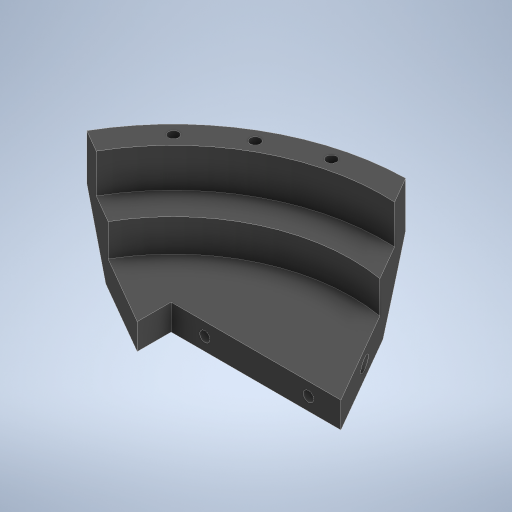
# Autodesk Inventor part: waist_side
Saved by Autodesk Inventor 2024.1 (Build 281209000, 209)
## iProperties
Created: 2024-02-14
Part Number: waist_side
Material: 一般
Document SubType Name: Modeling
Designer: hibik
Density: 1 g/cm^3
Appearance: 既定
Author: hibik
Autodesk Inventor part; units mm, degrees
ref_plane "YZ Plane" through (0, 0, 0) normal (1, 0, 0) x (0, 1, 0)
ref_plane "XZ Plane" through (0, 0, 0) normal (0, 1, 0) x (-1, 0, 0)
ref_plane "XY Plane" through (0, 0, 0) normal (0, 0, 1) x (1, 0, 0)
sketch "スケッチ1" plane through (0, 0, 0) normal (0, 1, 0) x (-1, 0, 0)
  circle A0 centre (0, 0) radius 27.5
  line L0 (13, 12.85) -> (-13, 12.85)
  line L1 (-13, 12.85) -> (-13, -12.85)
  line L2 (-13, -12.85) -> (13, -12.85)
  line L3 (13, -12.85) -> (13, 12.85)
  circle A1 centre (0, 0) radius 32.5
  circle A2 centre (0, 0) radius 36.5
  line L4 (0, 0) -> (18.4986, -32.0406)
  line L5 (0, 0) -> (31.6099, -18.25)
  line L6 (-13, -12.85) -> (0.651, -36.4942)
  line L7 (13.2, 12.8507) -> (13.2, -12.85)
  line L8 (13.2, -12.85) -> (13, -12.85)
  point P0 (13, 0)
  point P1 (0, 12.85)
  point P2 (13, -34.1065)
  point P3 (-13, -34.1065)
  point P4 (28.1458, -16.25)
  point P5 (13, -7.5056)
  point P6 (18.25, -31.6099)
  point P7 (16.25, -28.1458)
  point P8 (23.8157, -13.75)
  point P9 (-4.7839, -27.0807)
  point P10 (-1.6802, -32.4565)
  point P11 (13.2, -7.621)
  dimension "d0" = 55
  dimension "d1" = 12.85
  dimension "d2" = 26
  dimension "d3" = 5
  dimension "d4" = 4
  dimension "d11" = 60
  dimension "d12" = 30
  dimension "d16" = 0.2
  constraints: 18 end point, 4 coincident, 4 point on circle, 3 centre point, 3 parallel, 2 midpoint, 2 perpendicular, 1 concentric, 1 horizontal, 1 horizontal alignment, 1 vertical alignment
  measures "d0" diameter of A0
  measures "d1" distance from line of L2 point (0, 0)
  measures "d2" distance of L0.start L0.end
  measures "d3" radial gap between concentric circles of A1 A0
  measures "d4" radial gap between concentric circles of A2 A1
  measures "d11" angle of L2 L4
  measures "d12" angle of L5 L4
  measures "d16" distance between parallel lines of L7 L3
extrude "押し出し1" add sketch "スケッチ1" along normal blind 4 contours L6 L2 L4 A0 | A0 L4 A1 L6 | L5 A1 L4 A0 | A0 L4 L2 L8 L7 L5 | A1 L4 A2 L6 | L5 A2 L4 A1
extrude "押し出し2" add sketch "スケッチ1" along normal blind 9 contours A0 L4 A1 L6 | L5 A1 L4 A0
extrude "押し出し3" add sketch "スケッチ1" along normal blind 15 contours A1 L4 A2 L6 | L5 A2 L4 A1
chamfer "面取り1" distance 8 angle 45 1 edges at (-18.5312, 0, -31.4459)
sketch "スケッチ2" plane through (-13.2, 0, -12.85) normal (0, 0, 1) x (1, 0, 0)
  circle A0 centre (21.2, 2) radius 0.8 projected
  circle A1 centre (5.2, 2) radius 0.8 projected
  point P0 (13.2, 0)
extrude "押し出し4" cut sketch "スケッチ2" against normal through all
sketch "スケッチ4" plane through (0, 15, 0) normal (0, 1, 0) x (1, 0, 0)
  circle A0 centre (-24.3952, 24.3952) radius 0.8 projected
  line L0 (4.7839, 27.0807) -> (-0.651, 36.4942) projected
  arc A1 (-0.651, 36.4942) -> (-31.6099, 18.25) centre (0, 0) ccw projected
  line L1 (-31.6099, 18.25) -> (-23.8157, 13.75) projected
  arc A2 (4.7839, 27.0807) -> (-23.8157, 13.75) centre (0, 0) ccw projected
  circle A3 centre (-17.25, 29.8779) radius 0.8 projected
  circle A4 centre (-8.9293, 33.3244) radius 0.8 projected
  circle A5 centre (-24.3952, 24.3952) radius 0.8 projected
extrude "押し出し6" cut sketch "スケッチ4" against normal blind 4 contours A0 | A3 | A4
